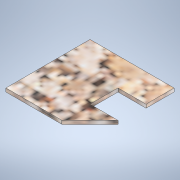
# Autodesk Inventor part: BetterTexas
Saved by Autodesk Inventor 2020 (Build 240168000, 168)
## iProperties
Created: 2019-10-27
Part Number: BetterTexas
Material: Generic
Document SubType Name: Modeling
Designer: Alex Zaccardelli
Density: 1 g/cm^3
Appearance: With Stone 2
Author: Alex Zaccardelli
Autodesk Inventor part; units mm, degrees
ref_plane "YZ Plane" through (0, 0, 0) normal (1, 0, 0) x (0, 1, 0)
ref_plane "XZ Plane" through (0, 0, 0) normal (0, 1, 0) x (-1, 0, 0)
ref_plane "XY Plane" through (0, 0, 0) normal (0, 0, 1) x (1, 0, 0)
sketch "Sketch1" plane through (0, 0, 0) normal (0, 1, 0) x (-1, 0, 0)
  line L0 (0, 0) -> (25.4, 0)
  line L1 (25.4, 0) -> (25.4, 25.4)
  line L2 (25.4, 25.4) -> (0, 25.4)
  line L3 (0, 25.4) -> (0, 0)
  line L4 (25.4, 25.4) -> (-12.7, 25.4)
  line L5 (0, 38.1) -> (25.4, 38.1)
  line L6 (25.4, 38.1) -> (25.4, 25.4)
  line L7 (0, 0) -> (-12.7, 0)
  line L8 (-12.7, 0) -> (-12.7, 12.7)
  line L9 (-12.7, 12.7) -> (0, 12.7)
  line L10 (0, 12.7) -> (0, 0)
  line L11 (-12.7, 25.4) -> (0, 38.1)
  dimension "d0" = 25.4
  dimension "d1" = 25.4
  dimension "d4" = 12.7
  dimension "d5" = 12.7
  constraints: 24 end point, 5 parallel, 3 horizontal, 2 perpendicular
  measures "d0" distance of L2.end L1.end
  measures "d1" distance of L1.end L0.end
  measures "d4" distance of L8.end L9.end
  measures "d5" distance of L7.end L8.end
extrude "Extrusion1" add sketch "Sketch1" along normal blind 1.6002
body "Solid1"
